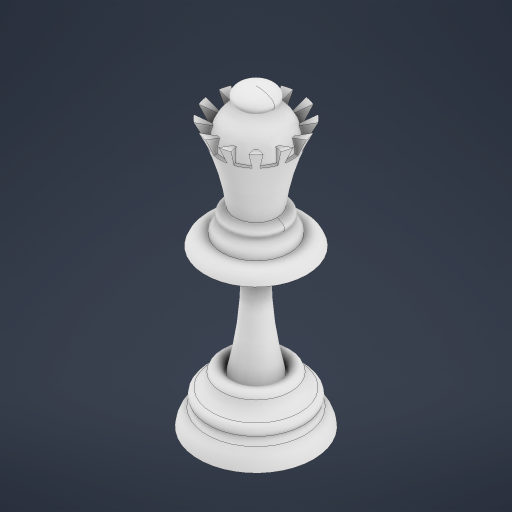
# Autodesk Inventor part: královna bílá
Saved by Autodesk Inventor 2023 (Build 270158000, 158)
## iProperties
Created: 2023-04-21
Part Number: královna bílá
Material: Generic
Document SubType Name: Modeling
Designer: X-DIABLO
Density: 1 g/cm^3
Appearance: Default
Author: X-DIABLO
Autodesk Inventor part; units mm, degrees
ref_plane "YZ Plane" through (0, 0, 0) normal (1, 0, 0) x (0, 1, 0)
ref_plane "XY Plane" through (0, 0, 0) normal (0, 0, 1) x (1, 0, 0)
sketch "Sketch1" plane through (0, 0, 0) normal (0, 0, 1) x (1, 0, 0)
  arc A0 (10.6154, 14.4572) -> (6.4844, 14.3615) centre (8.5595, 13.9943) ccw
  arc A1 (10.6154, 14.4572) -> (13.3879, 10.3297) centre (17.3221, 15.9672) ccw
  arc A2 (14.5003, 7.5665) -> (13.3879, 10.3297) centre (12.7286, 8.4588) ccw
  arc A3 (17.5, 0) -> (14.9429, 5.1854) centre (9.655, -0.6454) ccw
  arc A4 (14.5003, 7.5665) -> (14.9429, 5.1854) centre (16.2865, 6.6669) ccw
  line L0 (0, 0) -> (0, 90)
  arc A5 (0, 68.3151) -> (3.5629, 85.2337) centre (0, 77.1496) ccw
  line L1 (8.5295, 79.4509) -> (13.4988, 81.3102)
  arc A6 (13.4988, 81.3102) -> (6.4814, 58.3717) centre (71.721, 50.9562) ccw
  ellipse E0 centre (2.2798, 56.4869) end of major axis (8.7728, 56.4869) minor radius 2.4722 (6.9162, 54.7561) -> (6.4814, 58.3717) ccw
  arc A7 (10.3236, 50.9879) -> (6.9162, 54.7561) centre (6.8934, 51.3109) ccw
  line L2 (3.5729, 47.7401) -> (15.477, 47.7401)
  arc A8 (15.477, 47.7401) -> (10.3236, 50.9879) centre (10.9964, 46.3431) ccw
  arc A9 (3.5729, 47.7401) -> (6.4844, 14.3615) centre (113.6922, 40.5293) ccw
  line L3 (17.5, 0) -> (0, 0)
  arc A10 (3.5629, 85.2337) -> (0, 85.2337) centre (1.7814, 79.2825) ccw
  dimension "d0" = 2
  dimension "d1" = 90
  constraints: 23 point on circle, 11 centre point, 8 end point, 3 point on line, 3 tangent, 2 horizontal, 1 vertical, 4 other
  measures "d0" radius of A4
  measures "d1" distance of L0.start L0.end
revolve "Revolution1" add sketch "Sketch1" angle 360 about axis through (0, 0, 0) along (0, 1, 0)
ref_plane "Work Plane2" through (0, 85.984, 0) normal (0, 1, 0) x (-1, 0, 0)
sketch "Sketch2" plane through (0, 85.984, 0) normal (0, 1, 0) x (-1, 0, 0)
  circle A0 centre (0, 0) radius 13.4988 projected
  circle A1 centre (0, 0) radius 17.5 projected
  line L0 (2, 17.3853) -> (-2, 17.3853)
  line L1 (-2, 17.3853) -> (-2, -17.3853)
  line L2 (-2, -17.3853) -> (2, -17.3853)
  line L3 (2, -17.3853) -> (2, 17.3853)
  line L4 (0, 0) -> (-5.7122, 0) projected
  line L5 (2, 17.3853) -> (-2, -17.3853) construction
  line L6 (-2, 17.3853) -> (2, -17.3853) construction
  line L7 (22.5657, 2) -> (-22.5657, 2)
  line L8 (-22.5657, 2) -> (-22.5657, -2)
  line L9 (-22.5657, -2) -> (22.5657, -2)
  line L10 (22.5657, -2) -> (22.5657, 2)
  line L11 (22.5657, 2) -> (-22.5657, -2) construction
  line L12 (-22.5657, 2) -> (22.5657, -2) construction
  line L13 (-10.4247, 14.0561) -> (6.9606, -16.0561)
  line L14 (10.4247, -14.0561) -> (-6.9606, 16.0561)
  line L15 (-16.0561, 6.9606) -> (14.0561, -10.4247)
  line L16 (16.0561, -6.9606) -> (-14.0561, 10.4247)
  line L17 (-17.3853, -2) -> (17.3853, -2)
  line L18 (17.3853, 2) -> (-17.3853, 2)
  line L19 (-14.0561, -10.4247) -> (16.0561, 6.9606)
  line L20 (14.0561, 10.4247) -> (-16.0561, -6.9606)
  line L21 (-6.9606, -16.0561) -> (10.4247, 14.0561)
  line L22 (6.9606, 16.0561) -> (-10.4247, -14.0561)
  line L23 (2, -17.3853) -> (2, 17.3853)
  line L24 (-2, 17.3853) -> (-2, -17.3853)
  line L25 (10.4247, -14.0561) -> (-6.9606, 16.0561)
  line L26 (-10.4247, 14.0561) -> (6.9606, -16.0561)
  line L27 (16.0561, -6.9606) -> (-14.0561, 10.4247)
  line L28 (-16.0561, 6.9606) -> (14.0561, -10.4247)
  line L29 (17.3853, 2) -> (-17.3853, 2)
  line L30 (-17.3853, -2) -> (17.3853, -2)
  line L31 (14.0561, 10.4247) -> (-16.0561, -6.9606)
  line L32 (-14.0561, -10.4247) -> (16.0561, 6.9606)
  line L33 (6.9606, 16.0561) -> (-10.4247, -14.0561)
  line L34 (-6.9606, -16.0561) -> (10.4247, 14.0561)
  point P0 (-3.5629, 0)
  point P1 (2, -7.4641)
  point P2 (6.9606, -16.0561)
  point P3 (5.4641, -5.4641)
  point P4 (7.4641, -2)
  point P5 (7.4641, 2)
  point P6 (16.0561, 6.9606)
  point P7 (5.4641, 5.4641)
  point P8 (2, 7.4641)
  point P9 (-2, 7.4641)
  point P10 (-6.9606, 16.0561)
  point P11 (-5.4641, 5.4641)
  point P12 (-7.4641, 2)
  point P13 (-7.4641, -2)
  point P14 (-16.0561, -6.9606)
  point P15 (-5.4641, -5.4641)
  point P16 (-2, -7.4641)
  dimension "d4" = 4
  dimension "d5" = 4
  dimension "d8" = 360
  constraints: 68 end point, 4 midpoint, 4 parallel, 2 horizontal, 2 perpendicular, 1 point on circle, 73 other
  measures "d4" distance of L2.end L1.end
  measures "d5" distance of L8.end L7.end
extrude "Extrusion1" cut sketch "Sketch2" against normal blind 10 contours A0 L9 L16 L19 L7 | A0 L7 A1 L9 | L19 L7 L21 L20 A0 | A0 L20 A1 L19 | L7 L10 L9 A1 | L19 L16 L21 L7 | L16 A1 L15 A0 | A0 L15 L14 L9 L16 | L9 L14 L19 L16 | L21 L16 L3 L7 | L7 L3 L20 L21 | L19 L14 L21 L16 | L14 L15 L3 L9 | L9 L3 L19 L14 | L21 L20 L3 L22 A0 | A0 L22 A1 L21 | L7 L14 L20 L3 | L3 L16 L14 L7 | L21 L14 L3 L16 | L19 L3 L21 L14 | L14 A1 L13 A0 | A0 L13 L3 L15 L14 | L9 L21 L19 L3 | L3 L15 L21 L9 | L20 L14 L22 L3 | L3 L14 L16 | L14 L16 L7 | L7 L16 L20 L14 | L21 L3 L14 | L19 L21 L3 | L3 L13 L21 L15 | L21 L15 L19 L9 | L9 L19 L21 | L3 L22 L14 L1 A0 | A0 L1 L0 L3 | L20 L16 L22 L14 | L3 L21 L19 L9 L15 L13 L1 L22 L20 L7 L16 L14 | L7 L20 L16 | L3 L2 L1 A0 | A0 L1 L21 L13 L3 | L21 L13 L19 L15 | L19 L15 L9 | L22 L16 L1 L14 | L20 L7 L22 L16 | L20 L22 L7 | L21 L1 L19 L13 | L19 L13 L9 L15 | L9 L13 L15 | L14 L1 L16 L13 A0 | A0 L13 A1 L14 | L22 L7 L1 L16 | L22 L20 L1 L7 | L22 L1 L20 | L21 A1 L22 A0 | A0 L22 L19 L1 L21 | L19 L1 L9 L13 | L9 L1 L15 L13 | L15 L1 L13 | L1 L7 L13 L16 | L1 L20 L13 L7 | L1 L22 L13 L20 | L1 L4 L22 | L19 L22 L9 L1 | L9 L22 L15 L1 | L13 L4 L1 | L1 L15 L22 L13 | L16 L13 L7 L15 A0 | A0 L15 A1 L16 | L13 L20 L15 L7 | L13 L4 L20 | L22 L15 L4 | L19 A1 L20 A0 | A0 L20 L9 L22 L19 | L9 L20 L15 L22 | L15 L20 L9 A0 L7 | A0 L9 A1 L7 | A1 L9 L8 L7
sketch "Sketch3" plane through (0, 0, 0) normal (0, 0, 1) x (1, 0, 0)
  line L0 (-2, 75.984) -> (2, 75.984) projected
  circle A0 centre (0, 75.984) radius 10.0423
  line L1 (0, 86.0263) -> (0, 0)
  point P0 (0, 65.9417)
  constraints: 2 end point, 1 midpoint, 1 vertical, 3 other
revolve "Revolution2" add sketch "Sketch3" angle 360 about axis through (0, 86.0263, 0) along (0, -1, 0) picked at (6.6109, 75.2391) contours A0 L1
sketch "Sketch4" plane through (0, 0, 0) normal (0, 0, 1) x (1, 0, 0)
  point P0 (0, 0)
sketch "Sketch5" plane through (0, 0, 0) normal (0, 0, 1) x (1, 0, 0)
  ellipse E0 centre (0, 87.3248) end of major axis (5.7122, 87.3248) minor radius 2.6752 (3.5629, 85.2337) -> (0, 90) ccw
  line L0 (0, 0) -> (0, 90)
  line L1 (3.5629, 85.2337) -> (0, 85.2337)
  dimension "d14" = 90
  constraints: 4 end point, 1 perpendicular, 1 point on line, 1 vertical, 4 other
  measures "d14" distance of L0.start L0.end
revolve "Revolution3" add sketch "Sketch5" angle 360 about axis through (0, 0, 0) along (0, 1, 0)
body "Solid1"
